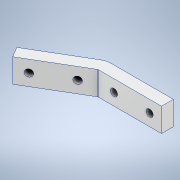
# Autodesk Inventor part: カウンター 取り付け根元曲げパーツ
Saved by Autodesk Inventor 2020.2 (Build 242310000, 310)
## iProperties
Created: 2020-05-03
Part Number: カウンター 取り付け根元曲げパーツ
Material: アルミニウム 6061
Document SubType Name: Modeling
Designer: mozar
Density: 2.7 g/cm^3
Appearance: アルミニウム - フラット
Mass: 6.95319 g
Surface Area: 18.6192 cm^2
Volume: 2.57526 cm^3
Author: mozar
Autodesk Inventor part; units mm, degrees
ref_plane "YZ Plane" through (0, 0, 0) normal (1, 0, 0) x (0, 1, 0)
ref_plane "XZ Plane" through (0, 0, 0) normal (0, 1, 0) x (-1, 0, 0)
ref_plane "XY Plane" through (0, 0, 0) normal (0, 0, 1) x (1, 0, 0)
sketch "スケッチ1" plane through (0, 0, 0) normal (0, 0, 1) x (1, 0, 0)
  circle A0 centre (-137.47813, 108.715013) radius 1.5
  circle A1 centre (-137.47813, 108.715013) radius 4
  circle A2 centre (-84.833891, 108.084965) radius 1.5
  circle A3 centre (-84.833891, 108.084965) radius 4
  arc A4 (-118.947299, 71.123436) -> (-117.73095, 71.382243) centre (-118.502117, 72.018876) ccw
  arc A5 (-114.600271, 73.907195) -> (-117.73095, 71.382243) centre (-110, 65) ccw
  arc A6 (-114.600271, 73.907195) -> (-114.089743, 75.041147) centre (-115.059151, 74.795694) ccw
  line L0 (-114.089743, 75.041147) -> (-119.33341, 95.750821)
  arc A7 (-119.33341, 95.750821) -> (-120.080809, 96.480412) centre (-120.302818, 95.505368) ccw
  arc A8 (-121.730917, 97.23053) -> (-120.080809, 96.480412) centre (-119.081767, 100.868113) ccw
  arc A9 (-121.730917, 97.23053) -> (-122.772044, 97.31398) centre (-122.319616, 96.422178) ccw
  line L1 (-122.772044, 97.31398) -> (-145.176978, 85.94755)
  arc A10 (-145.176978, 85.94755) -> (-145.169733, 84.160308) centre (-144.724551, 85.055748) ccw
  line L2 (-145.169733, 84.160308) -> (-118.947299, 71.123436)
  arc A11 (-111.181518, 75.777506) -> (-110.19287, 75.023145) centre (-110.212109, 76.022959) ccw
  arc A12 (-100.681376, 68.696468) -> (-110.19287, 75.023145) centre (-110, 65) ccw
  arc A13 (-100.681376, 68.696468) -> (-99.603497, 68.076257) centre (-99.751838, 69.065193) ccw
  line L3 (-99.603497, 68.076257) -> (-77.042446, 71.460414)
  arc A14 (-77.042446, 71.460414) -> (-76.670938, 73.303609) centre (-77.190786, 72.449351) ccw
  line L4 (-76.670938, 73.303609) -> (-114.637331, 96.407596)
  arc A15 (-114.637331, 96.407596) -> (-116.126588, 95.307885) centre (-115.15718, 95.553338) ccw
  line L5 (-116.126588, 95.307885) -> (-111.181518, 75.777506)
  circle A16 centre (-150.294817, 85.033166) radius 1.5
  arc A17 (-124.129325, 99.989384) -> (-123.581755, 100.878808) centre (-124.581752, 100.881185) ccw
  arc A18 (-114.594354, 100.531773) -> (-123.581755, 100.878808) centre (-119.081767, 100.868113) ccw
  arc A19 (-114.594354, 100.531773) -> (-114.117, 99.602773) centre (-113.597151, 100.457031) ccw
  line L6 (-114.117, 99.602773) -> (-73.405222, 74.828115)
  arc A20 (-73.405222, 74.828115) -> (-72.36076, 74.831033) centre (-72.885373, 75.682374) ccw
  arc A21 (-73.660486, 68.382589) -> (-72.36076, 74.831033) centre (-70, 71) ccw
  arc A22 (-73.660486, 68.382589) -> (-74.622268, 68.789879) centre (-74.473928, 67.800942) ccw
  line L7 (-74.622268, 68.789879) -> (-99.158476, 65.109447)
  arc A23 (-99.158476, 65.109447) -> (-100.006948, 64.200283) centre (-99.010135, 64.120511) ccw
  arc A24 (-119.754961, 67.311137) -> (-100.006948, 64.200283) centre (-110, 65) ccw
  arc A25 (-119.754961, 67.311137) -> (-120.282843, 68.437115) centre (-120.728025, 67.541674) ccw
  line L8 (-120.282843, 68.437115) -> (-147.085218, 81.762313)
  arc A26 (-147.085218, 81.762313) -> (-148.083283, 81.700131) centre (-147.5304, 80.866873) ccw
  arc A27 (-148.11038, 88.384022) -> (-148.083283, 81.700131) centre (-150.294817, 85.033166) ccw
  arc A28 (-148.11038, 88.384022) -> (-147.111844, 88.329935) centre (-147.564271, 89.221736) ccw
  line L9 (-147.111844, 88.329935) -> (-124.129325, 99.989384)
  circle A29 centre (-110, 65) radius 7.025
  circle A30 centre (-119.081767, 100.868113) radius 1.5
  circle A31 centre (-70, 71) radius 1.5
  line L10 (-330.399972, 95) -> (-110, 65)
  circle A32 centre (-156.443214, 91.162336) radius 4
  circle A33 centre (-136.470623, 92.209055) radius 4
  line L11 (0, 0) -> (-155.794817, 0)
  line L12 (-329.051247, 104.90863) -> (-108.651275, 74.90863)
  circle A34 centre (-156.443214, 91.162336) radius 9
  circle A35 centre (-136.470623, 92.209055) radius 6
  line L13 (-156.443214, 91.162336) -> (-136.470623, 92.209055)
  circle A36 centre (-110, 65) radius 65
  circle A37 centre (-191.443214, 91.162336) radius 5
  line L14 (-191.443214, 91.162336) -> (-156.443214, 91.162336)
  line L15 (-191.443214, 91.162336) -> (-206.443214, 91.162336)
  circle A38 centre (-206.443214, 91.162336) radius 5
  line L16 (-206.443214, 91.162336) -> (-221.443214, 91.162336)
  circle A39 centre (-221.443214, 91.162336) radius 5
  line L17 (-221.443214, 91.162336) -> (-236.443214, 91.162336)
  circle A40 centre (-236.443214, 91.162336) radius 5
  line L18 (-206.843214, 96.14631) -> (-157.163214, 100.133489)
  line L19 (-206.843214, 86.178361) -> (-157.163214, 82.191182)
  line L20 (-135.882319, 98.180143) -> (-155.560758, 100.118968)
  line L21 (-154.629369, 82.34701) -> (-135.261393, 86.332171)
  circle A41 centre (-206.443214, 91.162336) radius 1.5
  circle A42 centre (-191.443214, 91.162336) radius 1.5
  line L22 (-236.443214, 91.162336) -> (-191.443214, 91.162336) construction
  line L23 (-236.443214, 86.162336) -> (-191.443214, 86.162336)
  line L24 (-191.443214, 96.162336) -> (-236.443214, 96.162336)
  arc A43 (-236.443214, 96.162336) -> (-236.443214, 86.162336) centre (-236.443214, 91.162336) ccw
  arc A44 (-191.443214, 86.162336) -> (-191.443214, 96.162336) centre (-191.443214, 91.162336) ccw
  point P0 (-202.811763, 87.725395)
  point P1 (-169.324077, 83.167179)
  point P2 (-153.510113, 82.653698)
  point P3 (-153.460125, 82.587594)
  point P4 (-191.336809, 86.163468)
  point P5 (-192.881846, 86.373772)
  point P6 (-213.943214, 91.162336)
  dimension "d0" = 8
  dimension "d1" = 8
  dimension "d2" = 95
  dimension "d3" = 7.75125
  dimension "d4" = 10
  dimension "d5" = 18
  dimension "d6" = 12
  dimension "d7" = 20
  dimension "d8" = 3
  dimension "d9" = 130
  dimension "d10" = 10
  dimension "d11" = 35
  dimension "d12" = 15
  dimension "d13" = 10
  dimension "d14" = 15
  dimension "d15" = 10
  dimension "d16" = 15
  dimension "d17" = 10
  dimension "d18" = 3
  dimension "d19" = 3
  dimension "d20" = 10
  constraints: 60 point on circle, 52 end point, 45 centre point, 13 tangent, 8 coincident, 7 horizontal, 2 parallel, 1 concentric, 1 midpoint, 11 other
  measures "d0" diameter of A32
  measures "d1" diameter of A33
  measures "d2" distance from line of L11 L10.start
  measures "d3" angle of L11 L10
  measures "d4" distance between parallel lines of L10 L12
  measures "d5" diameter of A34
  measures "d6" diameter of A35
  measures "d7" distance of A32.centre A33.centre
  measures "d8" angle of L11 L13
  measures "d9" diameter of A36
  measures "d10" diameter of A37
  measures "d11" distance of L14.start L13.start
  measures "d12" distance of L14.start L15.end
  measures "d13" diameter of A38
  measures "d14" distance of L16.start L16.end
  measures "d15" diameter of A39
  measures "d16" distance of L17.start L17.end
  measures "d17" diameter of A40
  measures "d18" diameter of A41
  measures "d19" diameter of A42
  measures "d20" diameter of A44
extrude "押し出し1" add sketch "スケッチ1" against normal blind 5 contours A37 L12 | L12 A37 L15 A42 L14 | L23 A39 L12 A38 L19 | L19 A38 L23 | A37 L23 A38 L12 | L12 A38 L15 A37 | L14 A42 L15 A37 | A38 L12 | L23 A40 L17 L12 A39 | A39 L12 | L12 A38 L16 A41 L15 | L15 A38 L24 A37 | A42 L15 L14 | L14 L15 A42 | L24 A38 L18 | L18 A38 L16 A39 L24 | L12 A39 L16 A38 | A39 L17 L16 L12 | L12 L17 A39 | L15 A41 L16 A38 | A39 L16 L17 | A39 L17 L12 A40 L24 | L17 A40 L12 | A41 L16 L15 | L15 L16 A41
hole "穴1" at (-206.443214, 91.162336, 0) at (-191.443214, 91.162336, 0) direction (0, 0, -1) diameter 3 depth 12 tip angle 118
sketch "スケッチ2" plane through (0, 0, 0) normal (0, 0, 1) x (1, 0, 0)
  circle A0 centre (-206.443214, 91.162336) radius 1.5
  circle A1 centre (-191.443214, 91.162336) radius 1.5
  line L0 (-236.443214, 96.162336) -> (-191.443214, 96.162336)
  arc A2 (-191.443214, 86.162336) -> (-191.443214, 96.162336) centre (-191.443214, 91.162336) ccw
  line L1 (-191.443214, 86.162336) -> (-236.443214, 86.162336)
  arc A3 (-236.443214, 96.162336) -> (-236.443214, 86.162336) centre (-236.443214, 91.162336) ccw
  line L2 (-236.443214, 96.162336) -> (-239.443214, 96.162336)
  line L3 (-239.443214, 96.162336) -> (-239.443214, 86.162336)
  line L4 (-191.443214, 86.162336) -> (-236.443214, 86.162336)
  line L5 (-239.443214, 86.162336) -> (-236.443214, 86.162336)
  arc A4 (-191.443214, 86.162336) -> (-191.443214, 96.162336) centre (-191.443214, 91.162336) ccw
  line L6 (-191.443214, 96.162336) -> (-186.443214, 96.162336)
  line L7 (-186.443214, 96.162336) -> (-186.443214, 86.162336)
  line L8 (-186.443214, 86.162336) -> (-191.443214, 86.162336)
  line L9 (-191.443214, 96.162336) -> (-236.443214, 96.162336)
  line L10 (-236.443214, 86.162336) -> (-191.443214, 86.162336)
  arc A5 (-236.443214, 96.162336) -> (-236.443214, 86.162336) centre (-236.443214, 91.162336) ccw
  circle A6 centre (-234.443214, 91.162336) radius 5
  circle A7 centre (-219.443214, 91.162336) radius 5
  circle A8 centre (-206.443214, 91.162336) radius 1.5
  circle A9 centre (-206.443214, 91.162336) radius 5
  point P0 (0, 0)
  point P1 (-239.443214, 87.162336)
  point P2 (-186.443214, 91.162336)
  point P3 (-239.443214, 87.162336)
  point P4 (-239.443214, 95.162336)
  point P5 (-234.443214, 86.162336)
  point P6 (-234.443214, 96.162336)
  point P7 (-239.443214, 95.162336)
  dimension "d32" = 53
  dimension "d33" = 10
  dimension "d34" = 10
  dimension "d35" = 15
  dimension "d36" = 15
  dimension "d46" = 10
  constraints: 12 end point, 4 collinear, 4 tangent, 3 centre point, 2 perpendicular, 1 coincident
  measures "d32" distance between parallel lines of L3 L7
  measures "d33" diameter of A6
  measures "d34" diameter of A7
  measures "d35" distance of A1.centre A0.centre
  measures "d36" distance of A6.centre A7.centre
  measures "d46" diameter of A9
extrude "押し出し2" add sketch "スケッチ2" against normal blind 5 contours L0 A6 L3 A3 | A3 L3 L2 | A6 | A6 L1 A3 L3 | A3 L5 L3 | L6 L7 A2 | L7 L8 A2
hole "穴2" at (-234.443214, 91.162336, 0) at (-219.443214, 91.162336, 0) direction (0, 0, -1) diameter 3 depth 12 tip angle 118
sketch "スケッチ3" plane through (0, 0, 0) normal (0, 0, 1) x (1, 0, 0)
  circle A0 centre (-219.443214, 91.162336) radius 1.5
  line L0 (-186.443214, 96.162336) -> (-186.443214, 86.162336)
  line L1 (-186.443214, 86.162336) -> (-239.443214, 86.162336)
  line L2 (-239.443214, 86.162336) -> (-239.443214, 96.162336)
  line L3 (-239.443214, 96.162336) -> (-186.443214, 96.162336)
  circle A1 centre (-206.443214, 91.162336) radius 1.5
  circle A2 centre (-191.443214, 91.162336) radius 1.5
  line L4 (-186.443214, 96.162336) -> (-239.443214, 96.162336)
  line L5 (-212.943214, 96.162336) -> (-212.943214, 86.162336)
  line L6 (-239.443214, 86.162336) -> (-186.443214, 86.162336)
  circle A3 centre (-234.443214, 91.162336) radius 1.5
  point P0 (0, 0)
  constraints: 2 end point, 2 midpoint
bend part "曲げパーツ1" radius 1 angle 30.54 line through (-212.943214, 96.162336, 0) along (0, -1, 0) centre toward (0, 0, 1) moving side (-1, 0, 0) both sides no
equation "\"d36\" = d35"
